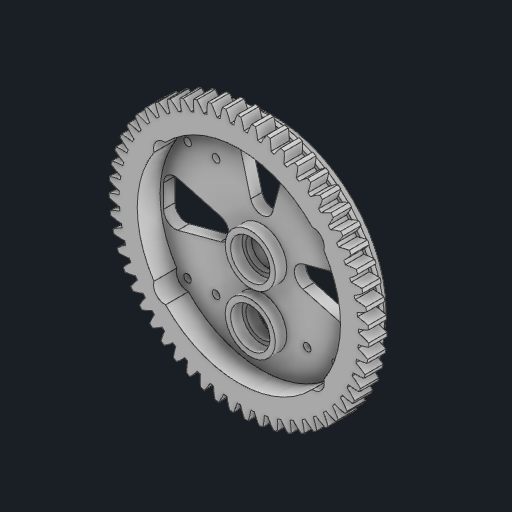
# Autodesk Inventor part: UpperWheelBracket
Saved by Autodesk Inventor 2023 (Build 270158000, 158)
## iProperties
Created: 2022-11-08
Part Number: UpperWheelBracket
Material: Generic
Document SubType Name: Modeling
Designer: izack
Density: 1 g/cm^3
Appearance: Default
Author: izack
## iProperties of the stored document UpperWheelBracket_3DPrint.ipt
Part Number: UpperWheelBracket_3DPrint
Material: Generic
Document SubType Name: Modeling
Designer: izack
Appearance: Default
Author: izack
Autodesk Inventor part; units mm, degrees
ref_plane "YZ Plane" through (0, 0, 0) normal (1, 0, 0) x (0, 1, 0)
ref_plane "XZ Plane" through (0, 0, 0) normal (0, 1, 0) x (-1, 0, 0)
sketch "Sketch1" plane through (0, 0, 0) normal (0, 0, 1) x (1, 0, 0)
  line L0 (90, 10) -> (0, 51.8) construction
  circle A0 centre (45, 30.9) radius 49.6166
  circle A1 centre (77.5, 5) radius 1.7 projected
  circle A2 centre (65, 5) radius 1.7 projected
  circle A3 centre (12.5, 5) radius 1.7 projected
  circle A4 centre (25, 5) radius 1.7 projected
  circle A5 centre (65, 5) radius 1.7 projected
  circle A6 centre (77.5, 5) radius 1.7 projected
  circle A7 centre (12.5, 5) radius 1.7 projected
  circle A8 centre (25, 5) radius 1.7 projected
  circle A9 centre (45, 30.9) radius 8.5
  circle A10 centre (45, 30.9) radius 44.6166
  circle A11 centre (12.5, 5) radius 5
  circle A12 centre (12.5, 5) radius 5
  circle A13 centre (77.5, 5) radius 5
  circle A14 centre (77.5, 5) radius 5
  line L1 (45, 30.9) -> (0.3834, 30.9) construction
  circle A15 centre (65, 56.8) radius 1.7
  circle A16 centre (77.5, 56.8) radius 1.7
  circle A17 centre (12.5, 56.8) radius 1.7
  circle A18 centre (25, 56.8) radius 1.7
  circle A19 centre (12.5, 56.8) radius 5
  circle A20 centre (77.5, 56.8) radius 5
  point P0 (0, 0)
  point P1 (0, 61.8)
  point P2 (0, 10)
  point P3 (90, 51.8)
  point P4 (90, 61.8)
  point P5 (90, 0)
  dimension "d4" = 5
  dimension "d1" = 17
  dimension "d5" = 10
  dimension "d6" = 10
  dimension "d7" = 10
  dimension "d8" = 10
  constraints: 11 centre point, 6 coincident, 6 symmetric about line, 4 end point, 1 horizontal, 1 horizontal alignment, 1 midpoint, 19 other
  measures "d1" diameter of A9
  measures "d5" diameter of A11
  measures "d6" diameter of A12
  measures "d7" diameter of A13
  measures "d8" diameter of A14
extrude "Extrusion2" add sketch "Sketch1" along normal blind 5 contours A0 | A9 | A10 A13 A11 A19 A20 | A20 A10 | A10 A20 | A13 A10 | A10 A13 | A19 A10 | A10 A19 | A11 A10 | A10 A11
sketch "Sketch2" plane through (45, 30.9, 5) normal (0, 0, 1) x (1, 0, 0)
  circle A0 centre (0, 0) radius 49.6166 projected
  circle A1 centre (0, 0) radius 44.6166 projected
  circle A2 centre (32.5, -25.9) radius 1.7 projected
  circle A3 centre (20, -25.9) radius 1.7 projected
  circle A4 centre (-20, -25.9) radius 1.7 projected
  circle A5 centre (-32.5, -25.9) radius 1.7 projected
  circle A6 centre (-32.5, -25.9) radius 1.7 projected
  circle A7 centre (-20, -25.9) radius 1.7 projected
  circle A8 centre (20, -25.9) radius 1.7 projected
  circle A9 centre (32.5, -25.9) radius 1.7 projected
  circle A10 centre (-32.5, -25.9) radius 5
  arc A11 (-30.8, -25.9) -> (-30.8, -25.9) centre (-32.5, -25.9) ccw projected
  circle A12 centre (-32.5, -25.9) radius 5
  arc A13 (34.2, -25.9) -> (34.2, -25.9) centre (34.0887, -24.2036) ccw
  arc A14 (34.2, -25.9) -> (34.2, -25.9) centre (32.5, -25.9) ccw projected
  circle A15 centre (32.5, -25.9) radius 5
  circle A16 centre (0, 0) radius 8.5
  circle A17 centre (0, 0) radius 13.5
  circle A18 centre (0, 0) radius 53.8666
  circle A19 centre (-32.5, -25.9) radius 1.7 projected
  line L0 (44.6166, 0) -> (-44.6166, 0) construction
  circle A20 centre (-32.5, 25.9) radius 5
  circle A21 centre (32.5, 25.9) radius 5
  circle A22 centre (0, 0) radius 60
  point P0 (-45, -30.9)
  point P1 (37.2963, -24.4873)
  point P2 (32.1934, -30.8906)
  point P3 (-32.1934, -30.8906)
  point P4 (-37.2963, -24.4873)
  point P5 (-32.1934, -30.8906)
  point P6 (-37.2963, -24.4873)
  point P7 (-37.2963, 24.4873)
  point P8 (-32.1934, 30.8906)
  point P9 (32.1934, 30.8906)
  point P10 (37.2963, 24.4873)
  dimension "d11" = 10
  dimension "d12" = 10
  dimension "d14" = 10
  dimension "d15" = 17
  dimension "d16" = 5
  dimension "d19" = 4.25
  dimension "d42" = 120
  constraints: 10 centre point, 5 coincident, 4 point on circle, 2 concentric, 2 end point, 2 symmetric about line, 1 horizontal, 2 other
  measures "d11" diameter of A10
  measures "d12" diameter of A12
  measures "d14" diameter of A15
  measures "d15" diameter of A16
  measures "d16" radial gap between concentric circles of A16 A17
  measures "d19" radial gap between concentric circles of A0 A18
  measures "d42" diameter of A22
extrude "Extrusion3" add sketch "Sketch2" along normal blind 10 contours A0 | A18
sketch "Sketch3" plane through (0, 0, 5) normal (0, 0, 1) x (1, 0, 0)
  circle A0 centre (45, 30.9) radius 53.8666 projected
  circle A1 centre (45, 30.9) radius 8.65
  circle A2 centre (45, 30.9) radius 11
  circle A3 centre (45, 30.9) radius 6.95
  arc A4 (82.2963, 6.4127) -> (7.7037, 6.4127) centre (45, 30.9) ccw construction
  arc A5 (14.2, 5) -> (14.2, 5) centre (12.5, 5) ccw construction
  arc A6 (79.2, 5) -> (79.2, 5) centre (77.5, 30.9029) ccw construction
  line L0 (12.5, 5) -> (77.5, 30.9029) construction
  line L1 (45, 30.9) -> (45, 17.9514) construction
  arc A7 (12.8066, 0.0094) -> (77.1934, 0.0094) centre (45, 30.9) ccw construction
  line L2 (45, 75.5166) -> (45, 17.9514) construction
  line L3 (40.1704, 48.9244) -> (35.1389, 67.7023)
  arc A8 (82.2963, 6.4127) -> (7.7037, 6.4127) centre (45, 30.9) ccw construction
  line L4 (49.8296, 48.9244) -> (54.8611, 67.7023)
  circle A9 centre (45, 30.9) radius 44.6166
  arc A10 (40.1704, 48.9244) -> (49.8296, 48.9244) centre (45, 50.2185) ccw
  arc A11 (40.1704, 48.9244) -> (49.8296, 48.9244) centre (45, 50.2185) ccw
  line L5 (39.9685, 73.9964) -> (50.0315, 73.9964)
  arc A12 (39.9685, 73.9964) -> (35.1389, 67.7023) centre (39.9685, 68.9964) ccw
  arc A13 (54.8611, 67.7023) -> (50.0315, 73.9964) centre (50.0315, 68.9964) ccw
  arc A14 (26.9756, 26.0704) -> (26.9756, 35.7296) centre (25.6815, 30.9) ccw
  line L6 (26.9756, 26.0704) -> (8.1977, 21.0389)
  arc A15 (1.9036, 25.8685) -> (8.1977, 21.0389) centre (6.9036, 25.8685) ccw
  line L7 (1.9036, 25.8685) -> (1.9036, 35.9315)
  arc A16 (8.1977, 40.7611) -> (1.9036, 35.9315) centre (6.9036, 35.9315) ccw
  line L8 (26.9756, 35.7296) -> (8.1977, 40.7611)
  arc A17 (49.8296, 12.8756) -> (40.1704, 12.8756) centre (45, 11.5815) ccw construction
  line L9 (49.8296, 12.8756) -> (54.8611, -5.9023) construction
  arc A18 (50.0315, -12.1964) -> (54.8611, -5.9023) centre (50.0315, -7.1964) ccw construction
  line L10 (50.0315, -12.1964) -> (39.9685, -12.1964) construction
  arc A19 (35.1389, -5.9023) -> (39.9685, -12.1964) centre (39.9685, -7.1964) ccw construction
  line L11 (40.1704, 12.8756) -> (35.1389, -5.9023) construction
  arc A20 (63.0244, 35.7296) -> (63.0244, 26.0704) centre (64.3185, 30.9) ccw
  line L12 (63.0244, 35.7296) -> (81.8023, 40.7611)
  arc A21 (88.0964, 35.9315) -> (81.8023, 40.7611) centre (83.0964, 35.9315) ccw
  line L13 (88.0964, 35.9315) -> (88.0964, 25.8685)
  arc A22 (81.8023, 21.0389) -> (88.0964, 25.8685) centre (83.0964, 25.8685) ccw
  line L14 (63.0244, 26.0704) -> (81.8023, 21.0389)
  circle A23 centre (45, 4.9) radius 6.95
  circle A24 centre (45, 4.9) radius 11
  circle A25 centre (45, 30.9) radius 60
  circle A26 centre (45, 4.9) radius 8.65
  line L15 (45, 17.9514) -> (45, -13.7166) construction
  point P0 (0, 0)
  point P1 (7.7037, 55.3873)
  point P2 (12.8066, 61.7906)
  point P3 (77.1934, 61.7906)
  point P4 (33.4524, 73.9964)
  point P5 (56.5476, 73.9964)
  point P6 (1.9036, 19.3524)
  point P7 (1.9036, 42.4476)
  point P8 (56.5476, -12.1964)
  point P9 (33.4524, -12.1964)
  point P10 (88.0964, 42.4476)
  point P11 (88.0964, 19.3524)
  dimension "d20" = 17.3
  dimension "d21" = 22
  dimension "d22" = 13.9
  dimension "d27" = 15
  dimension "d28" = 5
  dimension "d29" = 5
  dimension "d30" = 5
  dimension "d33" = 360
  dimension "d37" = 13.9
  dimension "d38" = 22
  dimension "d41" = 120
  dimension "d47" = 17.3
  dimension "d48" = 26
  constraints: 34 point on line, 32 end point, 31 point on circle, 21 centre point, 8 tangent, 7 coincident, 2 equal radius, 1 collinear, 1 horizontal, 1 midpoint, 1 symmetric about line, 82 other
  measures "d20" diameter of A1
  measures "d21" diameter of A2
  measures "d22" diameter of A3
  measures "d27" angle of L1 L3
  measures "d28" radius of A10
  measures "d29" radius of A11
  measures "d30" radius of A12
  measures "d37" diameter of A23
  measures "d38" diameter of A24
  measures "d41" diameter of A25
  measures "d47" diameter of A26
  measures "d48" distance of A1.centre A23.centre
extrude "Extrusion4" cut sketch "Sketch3" against normal blind 2.5 contours A3
extrude "Extrusion5" add sketch "Sketch3" along normal blind 5 contours A2 | A24
extrude "Extrusion6" cut sketch "Sketch3" against normal through all contours L3 A12 L5 A13 L4 A10 | L6 A15 L7 A16 L8 A14 | L12 A21 L13 A22 L14 A20 | A23
ref_plane "Work Plane1" through (0, 0, 7) normal (0, 0, 1) x (1, 0, 0)
sketch "Sketch4" plane through (0, 0, 7) normal (0, 0, 1) x (1, 0, 0)
  circle A0 centre (45, 30.9) radius 8.65 projected
  circle A1 centre (45, 30.9) radius 60
  circle A2 centre (45, 30.9) radius 53.8666 projected
  point P0 (0, 0)
  dimension "d44" = 120
  constraints: 1 centre point, 1 coincident
  measures "d44" diameter of A1
extrude "Extrusion8" add sketch "Sketch4" along normal up to surface (8 mm away) contours A1
spur gear teeth "Spur Gear1" teeth 55 pitch diameter 110 tip diameter 114 root diameter 105 face width 8 trims to tip circle yes start plane through (45, 30.9, 15) normal (0, 0, 1) x (1, 0, 0)
body "Solid2"
